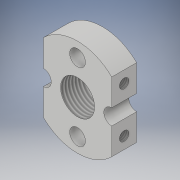
# Autodesk Inventor part: Part7
Saved by Autodesk Inventor 2019.1 (Build 231200000, 200)
## iProperties
Created: 2018-09-18
Part Number: Part7
Material: Generic
Document SubType Name: Modeling
Designer: drawing
Density: 1 g/cm^3
Appearance: Default
Author: drawing
Autodesk Inventor part; units mm, degrees
ref_plane "YZ Plane" through (0, 0, 0) normal (1, 0, 0) x (0, 1, 0)
ref_plane "XZ Plane" through (0, 0, 0) normal (0, 1, 0) x (-1, 0, 0)
ref_plane "XY Plane" through (0, 0, 0) normal (0, 0, 1) x (1, 0, 0)
sketch "Sketch1" plane through (0, 0, 0) normal (0, 0, 1) x (1, 0, 0)
  circle A0 centre (0, 0) radius 7.1437
  circle A1 centre (0, 0) radius 20.32
  dimension "d0" = 14.2875
  dimension "d1" = 40.64
  constraints: 2 centre point, 2 coincident
  measures "d0" diameter of A0
  measures "d1" diameter of A1
extrude "Extrusion1" add sketch "Sketch1" along normal blind 10.414
thread "Thread1" size "9/16-18 UNF" class "2B" standard "ANSI Unified Screw Threads" full length
sketch "Sketch2" plane through (0, 0, 10.414) normal (0, 0, 1) x (1, 0, 0)
  point P0 (0, 0)
  point P1 (0, 14.2875)
  dimension "d6" = 14.2875
  constraints: 1 vertical alignment
  measures "d6" distance of point (0, 14.287) point (0, 0)
hole "Hole1" at (0, 14.2875, 10.414) direction (0, 0, -1) diameter 6.604 depth 12.2936 tip angle 118
pattern_circular "Circular Pattern1" count 4 over 360 about axis through (0, 0, 0) along (0, 0, 1) of "Hole1"
sketch "Sketch3" plane through (0, 0, 10.414) normal (0, 0, 1) x (1, 0, 0)
  line L0 (-14.2875, -29.4711) -> (14.2875, -29.4711)
  line L1 (14.2875, -29.4711) -> (14.2875, 27.3802)
  line L2 (14.2875, 27.3802) -> (-14.2875, 27.3802)
  line L3 (-14.2875, 27.3802) -> (-14.2875, -29.4711)
  line L4 (-49.0321, -62.4929) -> (63.3318, -62.4929)
  line L5 (63.3318, -62.4929) -> (63.3318, 57.2179)
  line L6 (63.3318, 57.2179) -> (-49.0321, 57.2179)
  line L7 (-49.0321, 57.2179) -> (-49.0321, -62.4929)
  point P0 (0, 0)
  dimension "d17" = 28.575
  dimension "d18" = 14.2875
  constraints: 16 end point, 4 parallel, 2 horizontal, 2 perpendicular
  measures "d17" distance of L1.end L2.end
  measures "d18" distance from line of point (0, 0) L1
extrude "Extrusion2" cut sketch "Sketch3" against normal blind 10.414
sketch "Sketch4" plane through (14.2875, 3.302, 10.414) normal (1, 0, 0) x (0, 0, -1)
  line L0 (0, -6.604) -> (10.414, -6.604) projected
  line L1 (10.414, 0) -> (10.414, -6.604) projected
  line L2 (10.414, 0) -> (0, 0) projected
  line L3 (0, -6.604) -> (0, 0) projected
  line L4 (0, -3.302) -> (10.414, -3.302)
  point P0 (5.207, 6.223)
  point P1 (5.207, -3.302)
  point P2 (5.207, -12.827)
  dimension "d21" = 9.525
  dimension "d22" = 9.525
  constraints: 2 end point, 2 midpoint, 2 vertical alignment, 1 horizontal
  measures "d21" distance from line of point (5.207, 6.223) L4
  measures "d22" distance from line of L4 point (5.207, -12.827)
hole "Hole2" at (14.2875, 9.525, 5.207) at (14.2875, -9.525, 5.207) direction (-1, 0, 0) diameter 3.9624 depth 11.43 tip angle 118 thread size "10-32 UNF" class "2B" standard "ANSI Unified Screw Threads"
mirror "Mirror1" about plane through (0, 0, 0) normal (1, 0, 0) of "Hole2"
equation "\"d18\" = 0.5 * d17"
equation "\"d22\" = d21"
body "Solid1"
